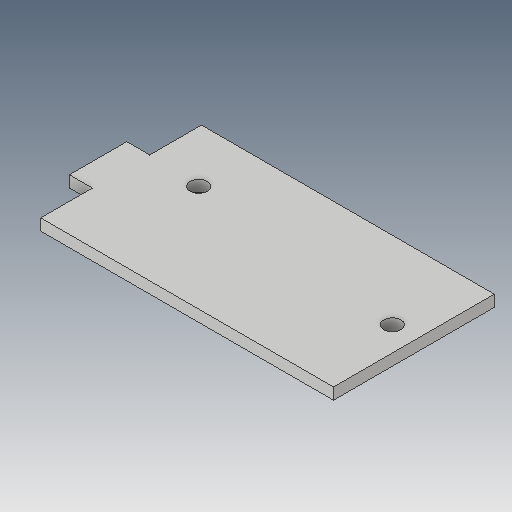
# Autodesk Inventor part: arm_2_microservo_case
Saved by Autodesk Inventor 2018 (Build 220112000, 112)
## iProperties
Created: 2018-02-08
Part Number: arm_2_microservo_case
Material: Genérico
Document SubType Name: Modeling
Designer: se_ma
Density: 1 g/cm^3
Appearance: Valor por defecto
Author: se_ma
Autodesk Inventor part; units mm, degrees
ref_plane "YZ Plane" through (0, 0, 0) normal (1, 0, 0) x (0, 1, 0)
ref_plane "XZ Plane" through (0, 0, 0) normal (0, 1, 0) x (-1, 0, 0)
ref_plane "XY Plane" through (0, 0, 0) normal (0, 0, 1) x (1, 0, 0)
sketch "Boceto1" plane through (0, 0, 0) normal (0, 1, 0) x (-1, 0, 0)
  line L0 (0, 0) -> (51, 0)
  line L1 (51, 0) -> (51, -28)
  line L2 (51, -28) -> (0, -28)
  line L3 (0, -28) -> (0, 0)
  line L4 (51, 0) -> (51, -18.5)
  line L5 (51, -18.5) -> (42, -18.5)
  circle A0 centre (42, -18.5) radius 1.5
  line L6 (0, 0) -> (0, -14.5)
  line L7 (0, -14.5) -> (4.25, -14.5)
  circle A1 centre (4.25, -14.5) radius 1.5
  line L8 (51, 0) -> (51, -14)
  line L9 (51, -14) -> (55, -14)
  line L10 (55, -14) -> (55, -9)
  line L11 (55, -9) -> (51, -9)
  line L12 (55, -14) -> (55, -19)
  line L13 (55, -19) -> (51, -19)
  dimension "d0" = 51
  dimension "d1" = 28
  dimension "d2" = 18.5
  dimension "d3" = 9
  dimension "d4" = 3
  dimension "d5" = 14.5
  dimension "d6" = 4.25
  dimension "d7" = 3
  dimension "d8" = 14
  dimension "d9" = 4
  dimension "d10" = 5
  dimension "d11" = 5
  constraints: 28 end point, 7 perpendicular, 6 point on line, 2 centre point, 2 coincident, 2 parallel, 1 horizontal
  measures "d0" distance of L1.end L2.end
  measures "d1" distance of L0.end L1.end
  measures "d2" distance of L0.end L4.end
  measures "d3" distance of L4.end L5.end
  measures "d4" diameter of A0
  measures "d5" distance of L0.start L6.end
  measures "d6" distance of L6.end L7.end
  measures "d7" diameter of A1
  measures "d8" distance of L0.end L8.end
  measures "d9" distance of L8.end L9.end
  measures "d10" distance of L9.end L10.end
  measures "d11" distance of L9.end L12.end
extrude "Extrusión1" add sketch "Boceto1" along normal blind 2
